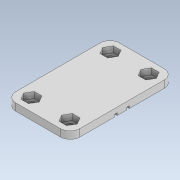
# Autodesk Inventor part: LED_COVER
Saved by Autodesk Inventor 2020 (Build 240168000, 168)
## iProperties
Created: 2020-08-12
Part Number: LED_COVER
Material: Generic
Document SubType Name: Modeling
Designer: Admin
Density: 1 g/cm^3
Appearance: Default
Author: Admin
Autodesk Inventor part; units mm, degrees
ref_plane "YZ Plane" through (0, 0, 0) normal (1, 0, 0) x (0, 1, 0)
ref_plane "XZ Plane" through (0, 0, 0) normal (0, 1, 0) x (-1, 0, 0)
ref_plane "XY Plane" through (0, 0, 0) normal (0, 0, 1) x (1, 0, 0)
sketch "Sketch1" plane through (0, 0, 0) normal (0, 1, 0) x (-1, 0, 0)
  line L0 (0, 0) -> (26.304, 0)
  line L1 (26.304, 0) -> (26.304, -38.6)
  line L2 (26.304, -38.6) -> (0, -38.6)
  line L3 (0, -38.6) -> (0, 0)
  dimension "d0" = 38.6
  dimension "d1" = 26.304
  constraints: 8 end point, 2 parallel, 1 horizontal, 1 perpendicular
  measures "d0" distance of L0.end L1.end
  measures "d1" distance of L1.end L2.end
extrude "Extrusion1" add sketch "Sketch1" along normal blind 3
sketch "Sketch2" plane through (0, 3, 0) normal (0, 1, 0) x (1, 0, 0)
  line L0 (-19.3893, 5.809) -> (-17.8016, 3.059)
  line L1 (-17.8016, 3.059) -> (-19.3893, 0.309)
  line L2 (-19.3893, 0.309) -> (-22.5647, 0.309)
  line L3 (-22.5647, 0.309) -> (-24.1524, 3.059)
  line L4 (-24.1524, 3.059) -> (-22.5647, 5.809)
  line L5 (-22.5647, 5.809) -> (-19.3893, 5.809)
  line L6 (-19.3893, 38.291) -> (-17.8016, 35.541)
  line L7 (-17.8016, 35.541) -> (-19.3893, 32.791)
  line L8 (-19.3893, 32.791) -> (-22.5647, 32.791)
  line L9 (-22.5647, 32.791) -> (-24.1524, 35.541)
  line L10 (-24.1524, 35.541) -> (-22.5647, 38.291)
  line L11 (-22.5647, 38.291) -> (-19.3893, 38.291)
  line L12 (-3.7393, 5.809) -> (-2.1516, 3.059)
  line L13 (-2.1516, 3.059) -> (-3.7393, 0.309)
  line L14 (-3.7393, 0.309) -> (-6.9147, 0.309)
  line L15 (-6.9147, 0.309) -> (-8.5024, 3.059)
  line L16 (-8.5024, 3.059) -> (-6.9147, 5.809)
  line L17 (-6.9147, 5.809) -> (-3.7393, 5.809)
  line L18 (-3.7393, 38.291) -> (-2.1516, 35.541)
  line L19 (-2.1516, 35.541) -> (-3.7393, 32.791)
  line L20 (-3.7393, 32.791) -> (-6.9147, 32.791)
  line L21 (-6.9147, 32.791) -> (-8.5024, 35.541)
  line L22 (-8.5024, 35.541) -> (-6.9147, 38.291)
  line L23 (-6.9147, 38.291) -> (-3.7393, 38.291)
  line L24 (-26.304, 0) -> (0, 0) projected
  line L25 (0, 38.6) -> (-26.304, 38.6) projected
  line L26 (0, 0) -> (0, 38.6) projected
  point P0 (-20.977, 3.059)
  point P1 (-20.977, 35.541)
  point P2 (-5.327, 3.059)
  point P3 (-5.327, 35.541)
  dimension "d4" = 5.5
  dimension "d6" = 5.5
  dimension "d7" = 5.5
  dimension "d8" = 5.5
  dimension "d9" = 32.482
  dimension "d10" = 32.482
  dimension "d11" = 15.65
  dimension "d12" = 0
  dimension "d13" = 0
  dimension "d14" = 3.059
  dimension "d15" = 5.327
  dimension "d16" = 15.65
  constraints: 48 end point, 4 parallel, 52 other
  measures "d4" distance between parallel lines of L1 L4
  measures "d6" distance between parallel lines of L7 L10
  measures "d7" distance between parallel lines of L13 L16
  measures "d8" distance between parallel lines of L19 L22
  measures "d9" distance of point (-20.977, 35.541) point (-20.977, 3.059)
  measures "d10" distance of point (-5.327, 35.541) point (-5.327, 3.059)
  measures "d11" distance of point (-5.327, 3.059) point (-20.977, 3.059)
  measures "d12" vertical distance of point (-5.327, 3.059) point (-20.977, 3.059)
  measures "d13" horizontal distance of point (-20.977, 3.059) point (-20.977, 35.541)
  measures "d14" distance from line of L24 point (-20.977, 3.059)
  measures "d15" distance from line of L26 point (-5.327, 3.059)
  measures "d16" distance of point (-5.327, 35.541) point (-20.977, 35.541)
extrude "Extrusion2" cut sketch "Sketch2" against normal blind 2.5
sketch "Sketch3" plane through (0, 0, 0) normal (1, 0, 0) x (0, 0, -1)
  line L0 (16.3, 1) -> (17.3, 1)
  line L1 (17.3, 1) -> (17.3, 0)
  line L2 (17.3, 0) -> (16.3, 0)
  line L3 (16.3, 0) -> (16.3, 1)
  line L4 (21.3, 1) -> (22.3, 1)
  line L5 (22.3, 1) -> (22.3, 0)
  line L6 (22.3, 0) -> (21.3, 0)
  line L7 (21.3, 0) -> (21.3, 1)
  line L8 (0, 0) -> (38.6, 0) projected
  line L9 (0, 0) -> (0, 3) projected
  dimension "d19" = 1
  dimension "d20" = 1
  dimension "d21" = 1
  dimension "d22" = 4
  dimension "d23" = 16.3
  constraints: 16 end point, 4 parallel, 3 point on line, 2 horizontal, 2 perpendicular
  measures "d19" distance of L4.start L4.end
  measures "d20" distance of L0.start L0.end
  measures "d21" distance of L2.end L0.start
  measures "d22" distance between parallel lines of L7 L1
  measures "d23" distance between parallel lines of L9 L3
extrude "Extrusion3" cut sketch "Sketch3" against normal blind 24
sketch "Sketch4" plane through (0, 3, 0) normal (0, 1, 0) x (1, 0, 0)
  circle A0 centre (-20.977, 3.059) radius 1.6
  circle A1 centre (-20.977, 35.541) radius 1.6
  circle A2 centre (-5.327, 35.541) radius 1.6
  circle A3 centre (-5.327, 3.059) radius 1.6
  line L0 (-19.3893, 0.309) -> (-22.5647, 0.309) projected
  line L1 (-3.7393, 0.309) -> (-6.9147, 0.309) projected
  line L2 (-22.5647, 38.291) -> (-19.3893, 38.291) projected
  line L3 (-6.9147, 38.291) -> (-3.7393, 38.291) projected
  line L4 (-24.1524, 3.059) -> (-22.5647, 5.809) projected
  line L5 (-22.5647, 32.791) -> (-24.1524, 35.541) projected
  line L6 (-3.7393, 5.809) -> (-2.1516, 3.059) projected
  line L7 (-3.7393, 38.291) -> (-2.1516, 35.541) projected
  point P0 (0, 0)
  dimension "d26" = 2.75
  dimension "d27" = 2.75
  dimension "d28" = 2.75
  dimension "d29" = 2.75
  dimension "d30" = 2.75
  dimension "d31" = 2.75
  dimension "d32" = 2.75
  dimension "d33" = 2.75
  dimension "d34" = 3.2
  dimension "d35" = 3.2
  dimension "d36" = 3.2
  dimension "d37" = 3.2
  constraints: 4 centre point
  measures "d26" distance from line of A0.centre L0
  measures "d27" distance from line of L1 A3.centre
  measures "d28" distance from line of L2 A1.centre
  measures "d29" distance from line of L3 A2.centre
  measures "d30" distance from line of A0.centre L4
  measures "d31" distance from line of L5 A1.centre
  measures "d32" distance from line of L6 A3.centre
  measures "d33" distance from line of L7 A2.centre
  measures "d34" diameter of A0
  measures "d35" diameter of A1
  measures "d36" diameter of A3
  measures "d37" diameter of A2
extrude "Extrusion4" cut sketch "Sketch4" against normal through all
sketch "Sketch5" plane through (0, 0, -38.6) normal (0, 0, -1) x (-1, 0, 0)
  line L0 (0, 0) -> (24, 0) projected
  line L1 (0, 0) -> (26.304, 0)
  line L2 (26.304, 0) -> (26.304, 3)
  line L3 (26.304, 3) -> (0, 3)
  line L4 (0, 3) -> (0, 0)
  constraints: 8 end point, 2 parallel, 1 coincident, 1 horizontal, 1 perpendicular
extrude "Extrusion5" add sketch "Sketch5" along normal blind 2
sketch "Sketch6" plane through (-26.304, 0, 0) normal (0, 0, 1) x (1, 0, 0)
  line L0 (2.304, 0) -> (26.304, 0) projected
  line L1 (26.304, 0) -> (0, 0)
  line L2 (0, 0) -> (0, 3)
  line L3 (0, 3) -> (26.304, 3)
  line L4 (26.304, 3) -> (26.304, 0)
  constraints: 8 end point, 2 parallel, 1 coincident, 1 horizontal, 1 perpendicular
extrude "Extrusion6" add sketch "Sketch6" along normal blind 2
fillet "Fillet1" radius 4 4 edges at (-26.304, 1.5, -40.6) (0, 1.5, -40.6) (0, 1.5, 2) (-26.304, 1.5, 2)
body "Solid1"
